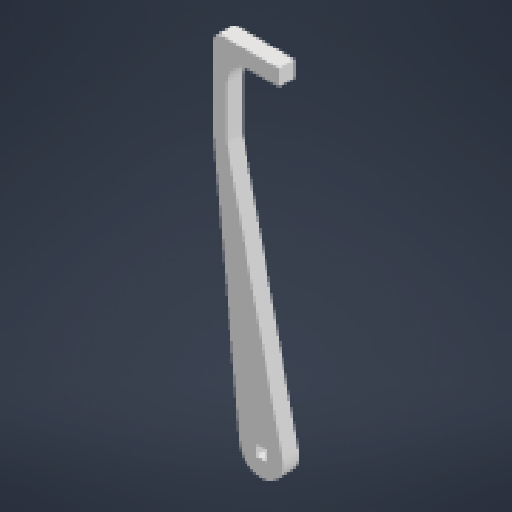
# Autodesk Inventor part: Arm
Saved by Autodesk Inventor 2025 (Build 290162000, 162)
## iProperties
Created: 2024-12-26
Part Number: Arm
Material: Типовые
Document SubType Name: Modeling
Designer: khrip
Density: 1 g/cm^3
Appearance: По умолчанию
Author: khrip
Autodesk Inventor part; units mm, degrees
ref_plane "YZ Plane" through (0, 0, 0) normal (1, 0, 0) x (0, 1, 0)
ref_plane "XZ Plane" through (0, 0, 0) normal (0, 1, 0) x (-1, 0, 0)
ref_plane "XY Plane" through (0, 0, 0) normal (0, 0, 1) x (1, 0, 0)
sketch "Эскиз1" plane through (0, 0, 0) normal (0, 0, 1) x (1, 0, 0)
  circle A0 centre (0.0899, -0.0505) radius 4 projected
  line L0 (-9.3607, -1.0179) -> (-20.8576, 111.2941)
  line L1 (-20.8576, 111.2941) -> (-20.8576, 149.3795)
  line L2 (-20.8576, 149.3795) -> (-6.2988, 149.3795)
  line L3 (7.9099, 149.3795) -> (-6.2988, 149.3795)
  line L4 (-14.8576, 142.2545) -> (7.9099, 142.2545)
  line L5 (-14.8576, 142.2545) -> (7.9099, 142.2545)
  line L6 (-14.8576, 109.9334) -> (-14.8576, 142.2545)
  line L7 (8.9694, 3.7673) -> (-14.8576, 109.9334)
  circle A1 centre (0.0899, -0.0505) radius 9.5
  line L8 (8.9285, 3.9495) -> (9.3593, 2.0299)
  line L9 (-2.25, -2.25) -> (2.25, -2.25)
  line L10 (2.25, -2.25) -> (2.25, 2.25)
  line L11 (2.25, 2.25) -> (-2.25, 2.25)
  line L12 (-2.25, 2.25) -> (-2.25, -2.25)
  line L13 (-2.25, -2.25) -> (2.25, 2.25) construction
  line L14 (2.25, -2.25) -> (-2.25, 2.25) construction
  line L15 (7.9099, 142.2545) -> (7.9099, 149.3795)
  point P0 (0, 0)
  dimension "d0" = 19
  dimension "d1" = 4.5
  dimension "d2" = 4.5
  constraints: 32 end point, 5 horizontal, 3 vertical, 2 midpoint, 2 parallel, 1 coincident, 1 perpendicular, 1 point on line, 14 other
  measures "d1" distance of L11.end L10.end
  measures "d2" distance of L10.end L9.end
extrude "Выдавливание1" add sketch "Эскиз1" along normal blind 7 contours A0 | L0 L1 L2 L3 L15 L4 L6 L7 L8 A1 | A1
fillet "Сопряжение1" radius 10 1 edges at (-14.8576, 142.2545, 3.5)
fillet "Сопряжение2" radius 4 1 edges at (-20.8576, 149.3795, 3.5)
